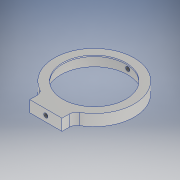
# Autodesk Inventor part: BSholder
Saved by Autodesk Inventor 2017 SP1 (Build 210196100, 196)
## iProperties
Created: 2015-08-04
Part Number: BSholder
Material: Generic
Document SubType Name: Modeling
Designer: Conor Mow-Lowry
Density: 1 g/cm^3
Appearance: Aluminum - Flat
Author: Conor Mow-Lowry
Autodesk Inventor part; units mm, degrees
ref_plane "YZ Plane" through (0, 0, 0) normal (1, 0, 0) x (0, 1, 0)
ref_plane "XY Plane" through (0, 0, 0) normal (0, 0, 1) x (1, 0, 0)
sketch "Sketch1" plane through (0, 0, 0) normal (0, 0, 1) x (1, 0, 0)
  circle A0 centre (0, 0) radius 25.4 construction
  circle A1 centre (0, 0) radius 26.4
  circle A2 centre (0, 0) radius 31.4
  line L0 (0, 0) -> (37.8275, -45.0811) construction
  line L1 (0, 0) -> (58.8492, 0) construction
  circle A3 centre (16.9696, -20.2236) radius 1
  line L2 (0, 0) -> (0, -31.4) construction
  circle A4 centre (-16.9696, -20.2236) radius 1
  dimension "d1" = 52.8
  dimension "d2" = 62.8
  dimension "d0" = 50.8
  dimension "d4" = 50
  constraints: 6 end point, 3 centre point, 3 coincident, 1 equal length, 1 horizontal, 1 point on line, 1 symmetric about line, 1 tangent, 1 vertical, 1 vertical alignment, 6 other
  measures "d0" diameter of A0
  measures "d4" angle of L0 L1
extrude "Extrusion1" add sketch "Sketch1" along normal blind 8 contours A4 A1 | A1 A4 | A3 A1 | A1 A3 | A2
fillet "Fillet1" radius 6 2 edges at (17.7233, -19.5664, 4) (16.1915, -20.8517, 4)
fillet_without_effect "Fillet2"
fillet "Fillet3" radius 6 2 edges at (-17.7233, -19.5664, 4) (-16.1915, -20.8517, 4)
fillet_without_effect "Fillet4"
sketch "Sketch2" plane through (0, 0, 8) normal (0, 0, 1) x (1, 0, 0)
  circle A0 centre (0, 0) radius 31.4 projected
  arc A1 (19.8973, -17.351) -> (-19.8973, -17.351) centre (0, 0) ccw projected
  circle A2 centre (0, 0) radius 24.9
  circle A3 centre (0, 0) radius 31.4
  dimension "d11" = 49.8
  constraints: 2 centre point, 2 coincident, 1 concentric
  measures "d11" diameter of A2
extrude "Extrusion2" add sketch "Sketch2" along normal blind 1
ref_plane "Work Plane1" through (0, 31.4, 0) normal (0, 1, 0) x (-1, 0, 0)
sketch "Sketch3" plane through (0, 31.4, 0) normal (0, 1, 0) x (-1, 0, 0)
  line L0 (-31.4, 0) -> (31.4, 0) projected
  point P0 (0, 0)
  point P1 (0, 4)
  dimension "d14" = 4
  measures "d14" distance from line of L0 point (0, 4)
hole "Hole1" at (0, 31.4, 4) direction (0, -1, 0) diameter 3.302 depth 12.3 tip angle 118 thread size "8-32 UNC" class "2B" standard "ANSI Unified Screw Threads"
sketch "Sketch4" plane through (0, 0, 0) normal (0, 0, -1) x (-1, 0, 0)
  circle A0 centre (0, 0) radius 31.4 projected
  arc A1 (-13.6322, -22.608) -> (13.6322, -22.608) centre (0, 0) ccw projected
  line L0 (-44.084, -38.1) -> (62.353, -38.1) construction
  line L1 (-12.7, -28.7171) -> (12.7, -28.7171)
  line L2 (12.7, -28.7171) -> (12.7, -38.1)
  line L3 (12.7, -38.1) -> (-12.7, -38.1)
  line L4 (-12.7, -38.1) -> (-12.7, -28.7171)
  line L5 (-12.7, -28.7171) -> (12.7, -38.1) construction
  line L6 (12.7, -28.7171) -> (-12.7, -38.1) construction
  line L7 (0, 0) -> (0, -74.2634) construction
  point P0 (0, -33.4085)
  point P1 (0, -33.4085)
  dimension "d22" = 38.1
  dimension "d23" = 25.4
  constraints: 16 end point, 3 midpoint, 2 horizontal, 2 parallel, 1 collinear, 1 perpendicular, 1 point on line, 1 vertical, 2 other
  measures "d22" distance from line of L0 point (0, 0)
  measures "d23" distance of L1.start L1.end
extrude "Extrusion3" add sketch "Sketch4" against normal blind 9 contours L1 A0 | A0 L2 L3 L4 picked at (-2.1634, -29.3854)
fillet "Fillet5" radius 6 1 edges at (12.7, -28.7171, 4.5)
fillet "Fillet6" radius 6 1 edges at (-12.7, -28.7171, 4.5)
sketch "Sketch5" plane through (-12.7, -38.1, 0) normal (0, -1, 0) x (1, 0, 0)
  line L0 (0, 9) -> (25.4, 9) projected
  line L1 (0, 0) -> (0, 9) projected
  line L2 (12.7, 0) -> (12.7, 9) construction
  line L3 (25.4, 9) -> (25.4, 0) construction
  line L4 (25.4, 4.5) -> (0, 4.5) construction
  point P0 (12.7, 4.5)
  constraints: 4 end point, 4 midpoint
hole "Hole2" at (0, -38.1, 4.5) direction (0, 1, 0) diameter 3.242 depth 13 tip angle 118 thread size "M4x0.7" class "6H" standard "ANSI Metric M Profile"
equation "\"d14\" = 0.5 * d5"
equation "\"d5\" = 8"
body "Solid1"
